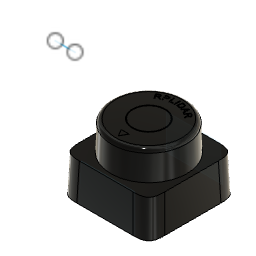
slamtec rplidar c1 (Autodesk Fusion 360 design; units mm, degrees)
Autodesk Fusion 360 part; units mm, degrees
sketch "Sketch1" plane through (0, 0, 0) normal (0, 0, 1) x (1, 0, 0)
  line L0 (27.8, -27.8) -> (-27.8, -27.8)
  line L1 (-27.8, -27.8) -> (-27.8, 27.8)
  line L2 (-27.8, 27.8) -> (27.8, 27.8)
  line L3 (27.8, 27.8) -> (27.8, -27.8)
  line L4 (27.8, -27.8) -> (-27.8, 27.8) construction
  line L5 (-27.8, -27.8) -> (27.8, 27.8) construction
  dimension "d1" = 55.6
  dimension "d2" = 55.6
  constraint horizontal L0
  constraint perpendicular L0 L1
  constraint parallel L0 L2
  constraint parallel L1 L3
  constraint coincident L4 origin
  constraint coincident L5 origin
  measures "d1" distance of L1.end L2.end
  measures "d2" distance of L0.end L1.end
sketch "Sketch2" plane through (0, 0, 0) normal (0, 1, 0) x (1, 0, 0)
  line L0 (-60.4372, -53.6913) -> (-48, -53.6913)
  constraint horizontal L0
extrude "Extrude1" add sketch "Sketch1" along normal blind 23.1 draft -2 makes body 1
fillet "Fillet1" radius 10 tangency weight 2 4 edges at (27.3967, -27.3967, 11.55) (-27.3967, -27.3967, 11.55) (27.3967, 27.3967, 11.55) (-27.3967, 27.3967, 11.55) on bodies 1
sketch "Sketch3" plane through (0, 0, 23.1) normal (0, 0, 1) x (-1, 0, 0)
  spline S0 degree 3 poles (26.9933, -16.9994) (26.9933, -18.9087) (26.8605, -20.6946) (26.1829, -23.0792) (25.8225, -23.8287) (24.9302, -24.9832) (24.4253, -25.4138) (23.1627, -26.1435) (22.3561, -26.4328) (20.1091, -26.8954) (18.6342, -26.9933) (16.9994, -26.9933) knots 0 0 0 0 0.572791 0.572791 0.932151 0.932151 1.250398 1.250398 1.609992 1.609992 2.076549 2.076549 2.076549 2.076549
  line L0 (26.9933, -16.9994) -> (26.9933, 16.9994)
  spline S1 degree 3 poles (16.9994, 26.9933) (18.9087, 26.9933) (20.6946, 26.8605) (23.0792, 26.1829) (23.8287, 25.8225) (24.9832, 24.9302) (25.4138, 24.4253) (26.1435, 23.1627) (26.4328, 22.3561) (26.8954, 20.1091) (26.9933, 18.6342) (26.9933, 16.9994) knots 0 0 0 0 0.572791 0.572791 0.932151 0.932151 1.250398 1.250398 1.609992 1.609992 2.076549 2.076549 2.076549 2.076549
  line L1 (16.9994, 26.9933) -> (-16.9994, 26.9933)
  spline S2 degree 3 poles (-26.9933, 16.9994) (-26.9933, 18.9087) (-26.8605, 20.6946) (-26.1829, 23.0792) (-25.8225, 23.8287) (-24.9302, 24.9832) (-24.4253, 25.4138) (-23.1627, 26.1435) (-22.3561, 26.4328) (-20.1091, 26.8954) (-18.6342, 26.9933) (-16.9994, 26.9933) knots 0 0 0 0 0.572791 0.572791 0.932151 0.932151 1.250398 1.250398 1.609992 1.609992 2.076549 2.076549 2.076549 2.076549
  line L2 (-26.9933, 16.9994) -> (-26.9933, -16.9994)
  spline S3 degree 3 poles (-16.9994, -26.9933) (-18.9087, -26.9933) (-20.6946, -26.8605) (-23.0792, -26.1829) (-23.8287, -25.8225) (-24.9832, -24.9302) (-25.4138, -24.4253) (-26.1435, -23.1627) (-26.4328, -22.3561) (-26.8954, -20.1091) (-26.9933, -18.6342) (-26.9933, -16.9994) knots 0 0 0 0 0.572791 0.572791 0.932151 0.932151 1.250398 1.250398 1.609992 1.609992 2.076549 2.076549 2.076549 2.076549
  line L3 (-16.9994, -26.9933) -> (16.9994, -26.9933)
  circle A0 centre (0, 0) radius 24
  dimension "d7" = 48
  constraint coincident A0.centre origin
  measures "d7" diameter of A0
extrude "Extrude2" add sketch "Sketch3" along normal blind 18.2 draft -2 contours A0 bodies 1
fillet "Fillet2" radius 2.5 1 edges at (21.7833, -8.4489, 41.3) on bodies 1
sketch "Sketch4" plane through (0, 27.7661, 0.9696) normal (0, 0.999391, 0.034899) x (-1, 0, 0)
  line L0 (16.9994, 22.1439) -> (17.8061, -0.9702)
  line L1 (16.9994, 22.1439) -> (-16.9994, 22.1439)
  line L2 (-17.8061, -0.9702) -> (-16.9994, 22.1439)
  line L3 (-17.8061, -0.9702) -> (17.8061, -0.9702)
sketch "Sketch5" plane through (0, 0, 41.3) normal (0, 0, 1) x (-1, 0, 0)
  circle A0 centre (0, 0) radius 20.9502
  circle A1 centre (0, 0) radius 10
  circle A2 centre (0, 0) radius 10.5
  dimension "d14" = 20
  dimension "d15" = 0.5
  constraint concentric A0 A1
  measures "d14" diameter of A1
extrude "Extrude3" cut sketch "Sketch5" against normal blind 0.5 contours A2 bodies 1
sketch "Sketch6" plane through (0, 0, 41.3) normal (0, 0, 1) x (-1, 0, 0)
  circle A0 centre (0, 0) radius 20.9502
  circle A1 centre (0, 0) radius 10.5
  circle A2 centre (0, 0) radius 16 construction
  dimension "d18" = 32
  dimension "d19" = 3.5
  text T0 "         RPLIDAR" font "Arial" height 3.5 align left spacing 1.1 along the path A2 letters at x, y, angle (-20.4368, 0.1883, 87.5677) (-20.3155, 2.2313, 81.8276) (-19.9904, 4.252, 76.0875) (-19.4649, 6.23, 70.3474) (-18.7442, 8.1456, 64.6074) (-17.8355, 9.9795, 58.8673) (-16.748, 11.7133, 53.1272) (-15.4925, 13.3296, 47.3871) (-14.0817, 14.8123, 41.647) (-12.3264, 16.3833, 32.017) (-8.1854, 18.7855, 18.98) (-3.9779, 20.0813, 7.3963) (-0.401, 20.4337, -0.7803) (1.9545, 20.4091, -10.4104) (6.6339, 19.3884, -23.4731) (10.7417, 17.4633, -36.5357)
  constraint coincident A0.centre A1.centre
  measures "d18" diameter of A2
extrude "Extrude4" cut sketch "Sketch6" against normal blind 1 text T0 bodies 1
sketch "Sketch7" plane through (0, 0, 41.3) normal (0, 0, 1) x (-1, 0, 0)
  circle A0 centre (0, 0) radius 10.5
  circle A1 centre (0, 0) radius 20.9502
  line L0 (9.7129, 14.6511) -> (8.7876, 13.4023)
  line L1 (8.7876, 13.4023) -> (8.4155, 13.678)
  line L2 (8.4155, 13.678) -> (10.4991, 16.4902)
  line L3 (10.4991, 16.4902) -> (11.746, 15.5664)
  spline S0 degree 3 poles (11.746, 15.5664) (11.8564, 15.4832) (12.0494, 15.3378) (12.1975, 15.1475) (12.2608, 15.0661) knots 0 0 0 0 0.041253 0.072059 0.072059 0.072059 0.072059
  spline S1 degree 3 poles (12.2608, 15.0661) (12.3005, 14.9895) (12.3816, 14.8334) (12.3778, 14.6574) (12.3759, 14.5678) knots 0 0 0 0 0.025447 0.051882 0.051882 0.051882 0.051882
  spline S2 degree 3 poles (12.3759, 14.5678) (12.3612, 14.4765) (12.3314, 14.2925) (12.23, 14.136) (12.1788, 14.0571) knots 0 0 0 0 0.027399 0.055273 0.055273 0.055273 0.055273
  spline S3 degree 3 poles (12.1788, 14.0571) (12.1007, 13.9674) (11.947, 13.791) (11.7219, 13.7274) (11.6112, 13.6962) knots 0 0 0 0 0.034845 0.068574 0.068574 0.068574 0.068574
  spline S4 degree 3 poles (11.6112, 13.6962) (11.4857, 13.6919) (11.2068, 13.6824) (10.9568, 13.8091) (10.8194, 13.8787) knots 0 0 0 0 0.037116 0.08243 0.08243 0.08243 0.08243
  spline S5 degree 3 poles (10.8194, 13.8787) (10.8475, 13.824) (10.8979, 13.7258) (10.9272, 13.6194) (10.9401, 13.5724) knots 0 0 0 0 0.018401 0.033001 0.033001 0.033001 0.033001
  spline S6 degree 3 poles (10.9401, 13.5724) (10.9543, 13.4772) (10.9842, 13.2773) (10.9761, 13.0753) (10.9718, 12.9695) knots 0 0 0 0 0.028796 0.060492 0.060492 0.060492 0.060492
  line L4 (10.9718, 12.9695) -> (10.8939, 11.8417)
  line L5 (10.8939, 11.8417) -> (10.4258, 12.1885)
  line L6 (10.4258, 12.1885) -> (10.4872, 13.0493)
  spline S7 degree 3 poles (10.4872, 13.0493) (10.4942, 13.1605) (10.5066, 13.3558) (10.506, 13.5515) (10.5057, 13.6358) knots 0 0 0 0 0.033406 0.058691 0.058691 0.058691 0.058691
  spline S8 degree 3 poles (10.5057, 13.6358) (10.5033, 13.699) (10.4991, 13.8107) (10.4684, 13.918) (10.4551, 13.9645) knots 0 0 0 0 0.018905 0.033364 0.033364 0.033364 0.033364
  spline S9 degree 3 poles (10.4551, 13.9645) (10.44, 14.0011) (10.4106, 14.0725) (10.3643, 14.1343) (10.3417, 14.1643) knots 0 0 0 0 0.011832 0.023063 0.023063 0.023063 0.023063
  spline S10 degree 3 poles (10.3417, 14.1643) (10.3168, 14.1888) (10.2552, 14.2493) (10.1858, 14.3007) (10.1445, 14.3313) knots 0 0 0 0 0.010461 0.025865 0.025865 0.025865 0.025865
  line L7 (10.1445, 14.3313) -> (9.7129, 14.6511)
  line L8 (-0.9374, 16.4291) -> (-0.8842, 16.0195)
  line L9 (-0.8842, 16.0195) -> (-3.0529, 15.7379)
  line L10 (-3.0529, 15.7379) -> (-3.5035, 19.2088)
  line L11 (-3.5035, 19.2088) -> (-3.0442, 19.2684)
  line L12 (-3.0442, 19.2684) -> (-2.6468, 16.2072)
  line L13 (-2.6468, 16.2072) -> (-0.9374, 16.4291)
  line L14 (-6.4139, 16.2187) -> (-5.9511, 14.8731)
  line L15 (-5.9511, 14.8731) -> (-6.3891, 14.7225)
  line L16 (-6.3891, 14.7225) -> (-7.5274, 18.0322)
  line L17 (-7.5274, 18.0322) -> (-6.2789, 18.4616)
  spline S11 degree 3 poles (-6.2789, 18.4616) (-6.1818, 18.4947) (-6.0131, 18.5521) (-5.8386, 18.5879) (-5.7646, 18.6031) knots 0 0 0 0 0.03075 0.053391 0.053391 0.053391 0.053391
  spline S12 degree 3 poles (-5.7646, 18.6031) (-5.6829, 18.6138) (-5.5279, 18.6342) (-5.3748, 18.6028) (-5.3024, 18.5879) knots 0 0 0 0 0.02451 0.046535 0.046535 0.046535 0.046535
  spline S13 degree 3 poles (-5.3024, 18.5879) (-5.235, 18.5634) (-5.0953, 18.5127) (-4.9855, 18.4123) (-4.9287, 18.3604) knots 0 0 0 0 0.021291 0.044125 0.044125 0.044125 0.044125
  spline S14 degree 3 poles (-4.9287, 18.3604) (-4.8747, 18.2997) (-4.7647, 18.176) (-4.7032, 18.0222) (-4.6719, 17.9438) knots 0 0 0 0 0.024182 0.049275 0.049275 0.049275 0.049275
  spline S15 degree 3 poles (-4.6719, 17.9438) (-4.636, 17.8057) (-4.5655, 17.5339) (-4.6519, 17.267) (-4.6944, 17.1357) knots 0 0 0 0 0.04185 0.082348 0.082348 0.082348 0.082348
  spline S16 degree 3 poles (-4.6944, 17.1357) (-4.7871, 17.0094) (-5.0072, 16.7097) (-5.3605, 16.5836) (-5.565, 16.5106) knots 0 0 0 0 0.046078 0.109338 0.109338 0.109338 0.109338
  line L18 (-5.565, 16.5106) -> (-6.4139, 16.2187)
  line L19 (6.0902, 15.9545) -> (5.3154, 15.1353)
  line L20 (5.3154, 15.1353) -> (4.8643, 15.3312)
  line L21 (4.8643, 15.3312) -> (7.4913, 18.0061)
  line L22 (7.4913, 18.0061) -> (7.949, 17.8074)
  line L23 (7.949, 17.8074) -> (7.8688, 14.0265)
  line L24 (7.8688, 14.0265) -> (7.3848, 14.2366)
  line L25 (7.3848, 14.2366) -> (7.4326, 15.3715)
  line L26 (7.4326, 15.3715) -> (6.0902, 15.9545)
  line L27 (0.5055, 19.4949) -> (0.4578, 15.9952)
  line L28 (0.4578, 15.9952) -> (-0.0053, 16.0016)
  line L29 (-0.0053, 16.0016) -> (0.0424, 19.5012)
  line L30 (0.0424, 19.5012) -> (0.5055, 19.4949)
  line L31 (-10.0851, 14.3974) -> (-9.2611, 13.0796)
  line L32 (-9.2611, 13.0796) -> (-9.6538, 12.834)
  line L33 (-9.6538, 12.834) -> (-11.5094, 15.8016)
  line L34 (-11.5094, 15.8016) -> (-10.1936, 16.6244)
  spline S17 degree 3 poles (-10.1936, 16.6244) (-10.0758, 16.6968) (-9.8699, 16.8232) (-9.6386, 16.8914) (-9.5397, 16.9206) knots 0 0 0 0 0.041253 0.072059 0.072059 0.072059 0.072059
  spline S18 degree 3 poles (-9.5397, 16.9206) (-9.4539, 16.9296) (-9.279, 16.948) (-9.1166, 16.8801) (-9.0338, 16.8455) knots 0 0 0 0 0.025447 0.051882 0.051882 0.051882 0.051882
  spline S19 degree 3 poles (-9.0338, 16.8455) (-8.9543, 16.7985) (-8.7938, 16.7035) (-8.6853, 16.5519) (-8.6306, 16.4754) knots 0 0 0 0 0.027399 0.055273 0.055273 0.055273 0.055273
  spline S20 degree 3 poles (-8.6306, 16.4754) (-8.5757, 16.3699) (-8.4676, 16.1623) (-8.4908, 15.9296) (-8.5022, 15.8152) knots 0 0 0 0 0.034845 0.068574 0.068574 0.068574 0.068574
  spline S21 degree 3 poles (-8.5022, 15.8152) (-8.5441, 15.6967) (-8.6372, 15.4337) (-8.8465, 15.2473) (-8.9616, 15.1449) knots 0 0 0 0 0.037116 0.08243 0.08243 0.08243 0.08243
  spline S22 degree 3 poles (-8.9616, 15.1449) (-8.9004, 15.1511) (-8.7905, 15.1621) (-8.6809, 15.1504) (-8.6324, 15.1453) knots 0 0 0 0 0.018401 0.033001 0.033001 0.033001 0.033001
  spline S23 degree 3 poles (-8.6324, 15.1453) (-8.5386, 15.1237) (-8.3416, 15.0784) (-8.1566, 14.997) (-8.0596, 14.9543) knots 0 0 0 0 0.028796 0.060492 0.060492 0.060492 0.060492
  line L35 (-8.0596, 14.9543) -> (-7.0384, 14.4694)
  line L36 (-7.0384, 14.4694) -> (-7.5323, 14.1605)
  line L37 (-7.5323, 14.1605) -> (-8.3111, 14.5324)
  spline S24 degree 3 poles (-8.3111, 14.5324) (-8.412, 14.5796) (-8.5893, 14.6625) (-8.7716, 14.7335) (-8.8502, 14.7641) knots 0 0 0 0 0.033406 0.058691 0.058691 0.058691 0.058691
  spline S25 degree 3 poles (-8.8502, 14.7641) (-8.9099, 14.785) (-9.0154, 14.8219) (-9.1265, 14.8325) (-9.1746, 14.8372) knots 0 0 0 0 0.018905 0.033364 0.033364 0.033364 0.033364
  spline S26 degree 3 poles (-9.1746, 14.8372) (-9.2142, 14.8365) (-9.2915, 14.8353) (-9.3659, 14.8147) (-9.4021, 14.8047) knots 0 0 0 0 0.011832 0.023063 0.023063 0.023063 0.023063
  spline S27 degree 3 poles (-9.4021, 14.8047) (-9.434, 14.7905) (-9.5128, 14.7553) (-9.586, 14.7095) (-9.6296, 14.6822) knots 0 0 0 0 0.010461 0.025865 0.025865 0.025865 0.025865
  line L38 (-9.6296, 14.6822) -> (-10.0851, 14.3974)
  spline S28 degree 3 poles (3.3305, 15.7166) (3.2417, 15.7152) (3.0529, 15.7123) (2.8666, 15.743) (2.7679, 15.7593) knots 0 0 0 0 0.026582 0.056522 0.056522 0.056522 0.056522
  line L39 (2.7679, 15.7593) -> (1.5257, 15.9875)
  line L40 (1.5257, 15.9875) -> (2.1582, 19.4299)
  line L41 (2.1582, 19.4299) -> (3.344, 19.212)
  spline S29 degree 3 poles (3.344, 19.212) (3.4622, 19.1898) (3.6677, 19.1511) (3.8643, 19.0802) (3.9478, 19.0501) knots 0 0 0 0 0.036013 0.062601 0.062601 0.062601 0.062601
  spline S30 degree 3 poles (3.9478, 19.0501) (4.037, 19.0063) (4.2108, 18.921) (4.343, 18.7796) (4.4073, 18.7108) knots 0 0 0 0 0.029523 0.05755 0.05755 0.05755 0.05755
  spline S31 degree 3 poles (4.4073, 18.7108) (4.4775, 18.6119) (4.6205, 18.4103) (4.6767, 18.1695) (4.7053, 18.0468) knots 0 0 0 0 0.036002 0.073401 0.073401 0.073401 0.073401
  spline S32 degree 3 poles (4.7053, 18.0468) (4.7217, 17.9129) (4.7562, 17.6317) (4.7136, 17.3514) (4.6913, 17.2046) knots 0 0 0 0 0.040277 0.084581 0.084581 0.084581 0.084581
  spline S33 degree 3 poles (4.6913, 17.2046) (4.6657, 17.0812) (4.6169, 16.8472) (4.5186, 16.6294) (4.4721, 16.5264) knots 0 0 0 0 0.037674 0.07147 0.07147 0.07147 0.07147
  spline S34 degree 3 poles (4.4721, 16.5264) (4.4238, 16.4379) (4.3331, 16.2715) (4.2049, 16.1322) (4.1449, 16.067) knots 0 0 0 0 0.030109 0.056583 0.056583 0.056583 0.056583
  spline S35 degree 3 poles (4.1449, 16.067) (4.086, 16.0143) (3.9731, 15.9133) (3.8377, 15.8451) (3.7729, 15.8125) knots 0 0 0 0 0.023585 0.04525 0.04525 0.04525 0.04525
  spline S36 degree 3 poles (3.7729, 15.8125) (3.705, 15.788) (3.5619, 15.7363) (3.4102, 15.7234) (3.3305, 15.7166) knots 0 0 0 0 0.021547 0.045443 0.045443 0.045443 0.045443
  line L42 (-0.164, -10.4987) -> (-0.164, -21.9983) construction
  line L43 (-0.164, -19.1216) -> (2.336, -14.7915)
  line L44 (-0.164, -19.1216) -> (4.836, -19.1216) construction
  line L45 (-0.164, -19.1216) -> (-2.664, -14.7915)
  line L46 (-2.664, -14.7915) -> (2.336, -14.7915)
  dimension "d22" = 5
  dimension "d23" = 60
  constraint coincident A0 L42.start
  constraint vertical L42
  constraint horizontal L44
  constraint coincident L42 L43.start
  constraint symmetric L42 L43.start L44.start
  constraint symmetric L42 L43.end L45.end
  measures "d22" distance of L43.start L43.end
  measures "d23" angle of L43 L44
extrude "Extrude5" add sketch "Sketch7" along normal blind 0.1 contours L43 L45 L46 bodies 1
sketch "Sketch8" plane through (0, -27.7661, 0.9696) normal (0, -0.999391, 0.034899) x (1, 0, 0)
  line L0 (-17.8061, -0.9702) -> (-16.9994, 22.1439)
  line L1 (-17.8061, -0.9702) -> (17.8061, -0.9702)
  line L2 (16.9994, 22.1439) -> (17.8061, -0.9702)
  line L3 (16.9994, 22.1439) -> (-16.9994, 22.1439)
move_body "Move1" bodies 1 to x (-1, 0, 0) y (0, -1, 0) z (0, 0, 1) at (-55.6146, -55.6146, 0)
move_body "Move2" bodies 1 to x (1, 0, 0) y (0, 1, 0) z (0, 0, 1) at (55, 0, 0)
move_body "Move3" bodies 1 to x (1, 0, 0) y (0, 1, 0) z (0, 0, 1) at (0, 55, 0)
sketch "Sketch9" plane through (0, 27.7661, 0.9696) normal (0, 0.999391, 0.034899) x (-1, 0, 0)
  line L0 (2.6616, 6.9571) -> (-3.3384, 6.9571)
  line L1 (-5.3384, 4.9571) -> (-5.3384, -1.0429)
  line L2 (-5.3384, -1.0429) -> (4.6616, -1.0429)
  line L3 (4.6616, -1.0429) -> (4.6616, 4.9571)
  line L4 (4.6616, 6.9571) -> (-5.3384, -1.0429) construction
  line L5 (-5.3384, 6.9571) -> (4.6616, -1.0429) construction
  arc A0 (-3.3384, 6.9571) -> (-5.3384, 4.9571) centre (-3.3384, 4.9571) ccw
  arc A1 (4.6616, 4.9571) -> (2.6616, 6.9571) centre (2.6616, 4.9571) ccw
  point P0 (-0.3384, 2.9571)
  dimension "d26" = 10
  dimension "d27" = 8
  dimension "d28" = 2
  constraint horizontal L0
  constraint perpendicular L0 L1
  constraint parallel L0 L2
  constraint parallel L1 L3
  constraint coincident L4 P0
  constraint coincident L5 P0
  constraint coincident L5.start L0
  constraint coincident L5.start L1
  constraint tangent L0 A0
  constraint tangent L1 A0
  constraint coincident L4.start L0
  constraint coincident L4.start L3
  constraint tangent L0 A1
  constraint tangent L3 A1
  constraint equal A0 A1
  measures "d26" distance of L1.end L2.end
  measures "d27" distance of L5.start L1.end
  measures "d28" radius of A0
extrude "Extrude6" add sketch "Sketch9" along normal blind 5 separate body makes body 2
fillet "Fillet3" radius 0.5 6 edges at (0.3384, 32.7995, 0.1019) (-4.6616, 32.6948, 3.1) (-4.0758, 32.5407, 7.5116) (0.3384, 32.5203, 8.097) (4.7526, 32.5407, 7.5116) (5.3384, 32.6948, 3.1) on bodies 2
